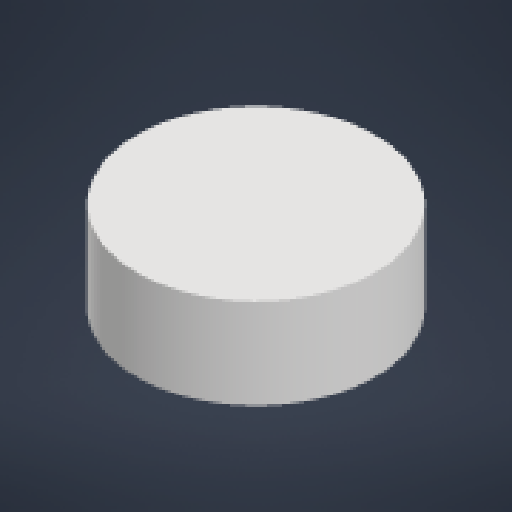
# Autodesk Inventor part: GGT
Saved by Autodesk Inventor 2024.2 (Build 282272000, 272)
## iProperties
Created: 2024-03-10
Part Number: GGT
Material: Generic
Document SubType Name: Modeling
Designer: warm
Density: 1 g/cm^3
Appearance: Default
Author: warm
Autodesk Inventor part; units mm, degrees
ref_plane "YZ Plane" through (0, 0, 0) normal (1, 0, 0) x (0, 1, 0)
ref_plane "XZ Plane" through (0, 0, 0) normal (0, 1, 0) x (-1, 0, 0)
ref_plane "XY Plane" through (0, 0, 0) normal (0, 0, 1) x (1, 0, 0)
sketch "Sketch4" plane through (0, 0, 0) normal (1, 0, 0) x (0, 1, 0)
  line L0 (0, 0) -> (0, -26.0096)
  line L1 (0, 0) -> (33.46, 0)
  line L2 (33.46, 0) -> (33.46, -26.0096)
  line L3 (33.46, -26.0096) -> (0, -26.0096)
  line L4 (35.286, -25.908) -> (35.1766, -0.1801)
  arc A0 (35.286, -25.908) -> (35.2799, -24.4856) centre (35.283, -25.1968) ccw
  arc A1 (35.2795, -24.384) -> (35.2735, -22.9616) centre (35.2765, -23.6728) ccw
  arc A2 (35.273, -22.86) -> (35.267, -21.4376) centre (35.27, -22.1488) ccw
  arc A3 (35.2665, -21.336) -> (35.2605, -19.9137) centre (35.2635, -20.6248) ccw
  arc A4 (35.2601, -19.8121) -> (35.254, -18.3897) centre (35.257, -19.1009) ccw
  arc A5 (35.2536, -18.2881) -> (35.2475, -16.8657) centre (35.2506, -17.5769) ccw
  arc A6 (35.2471, -16.7641) -> (35.2411, -15.3417) centre (35.2441, -16.0529) ccw
  arc A7 (35.2406, -15.2401) -> (35.2346, -13.8177) centre (35.2376, -14.5289) ccw
  arc A8 (35.2342, -13.7161) -> (35.2281, -12.2937) centre (35.2311, -13.0049) ccw
  arc A9 (35.2277, -12.1921) -> (35.2216, -10.7697) centre (35.2247, -11.4809) ccw
  arc A10 (35.2212, -10.6681) -> (35.2152, -9.2458) centre (35.2182, -9.9569) ccw
  arc A11 (35.2147, -9.1442) -> (35.2087, -7.7218) centre (35.2117, -8.433) ccw
  arc A12 (35.2083, -7.6202) -> (35.2022, -6.1978) centre (35.2052, -6.909) ccw
  arc A13 (35.2018, -6.0962) -> (35.1957, -4.6738) centre (35.1988, -5.385) ccw
  arc A14 (35.1953, -4.5722) -> (35.1893, -3.1498) centre (35.1923, -3.861) ccw
  arc A15 (35.1888, -3.0482) -> (35.1828, -1.6258) centre (35.1858, -2.337) ccw
  arc A16 (35.1824, -1.5242) -> (35.1763, -0.1018) centre (35.1793, -0.813) ccw
  line L5 (35.1763, -0.1018) -> (33.46, -0.1018)
  line L6 (35.286, -25.908) -> (33.46, -25.908)
  point P0 (35.2799, -24.4856)
  point P1 (35.2735, -22.9616)
  point P2 (35.267, -21.4376)
  point P3 (35.2605, -19.9137)
  point P4 (35.254, -18.3897)
  point P5 (35.2536, -18.2881)
  point P6 (35.2475, -16.8657)
  point P7 (35.2411, -15.3417)
  point P8 (35.2406, -15.2401)
  point P9 (35.2346, -13.8177)
  point P10 (35.2342, -13.7161)
  point P11 (35.2281, -12.2937)
  point P12 (35.2277, -12.1921)
  point P13 (35.2216, -10.7697)
  point P14 (35.2152, -9.2458)
  point P15 (35.2087, -7.7218)
  point P16 (35.2083, -7.6202)
  point P17 (35.2022, -6.1978)
  point P18 (35.2018, -6.0962)
  point P19 (35.1957, -4.6738)
  point P20 (35.1953, -4.5722)
  point P21 (35.1893, -3.1498)
  point P22 (35.1888, -3.0482)
  point P23 (35.1828, -1.6258)
  point P24 (35.1824, -1.5242)
  dimension "d12" = 26.0096
  dimension "d13" = 33.46
  dimension "d14" = 1.8288
  dimension "d18" = 1.524
  dimension "d25" = 0.7112
  dimension "d26" = 0.243
  dimension "d27" = 0.1016
  dimension "d28" = 0
  constraints: 34 point on circle, 17 centre point, 16 equal radius, 12 end point, 4 perpendicular, 2 point on line, 1 horizontal, 1 vertical, 52 other
  measures "d12" distance of L0.start L0.end
  measures "d13" distance of L0.start L1.end
  measures "d14" distance of L2.end L6.start
  measures "d18" distance of A0.centre A1.centre
  measures "d25" radius of A0
  measures "d27" vertical distance of L6.start L2.end
revolve "Revolution1" add sketch "Sketch4" angle 360 about axis through (0, 0, 0) along (0, 0, -1) contours L5 A16 L4 L6 L2 | L4 A0 | A15 L4 | L4 A1 | A14 L4 | L4 A2 | A13 L4 | L4 A3 | A12 L4 | L4 A4 | A11 L4 | L4 A5 | A10 L4 | L4 A6 | A9 L4 | L4 A7 | A8 L4
body "Solid3"
